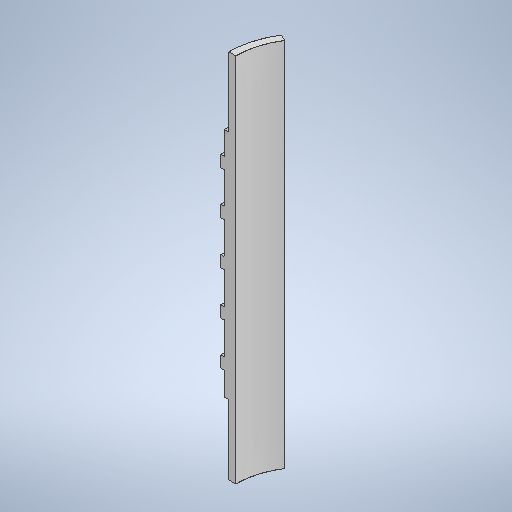
# Autodesk Inventor part: Bumper_V1
Saved by Autodesk Inventor 2025.2 (Build 292293000, 293)
## iProperties
Created: 2026-01-12
Part Number: Bumper_V1
Material: Generisch
Document SubType Name: Modeling
Designer: gassl
Density: 1 g/cm^3
Appearance: Vorgabe
Author: gassl
Autodesk Inventor part; units mm, degrees
ref_plane "YZ Plane" through (0, 0, 0) normal (1, 0, 0) x (0, 1, 0)
ref_plane "XZ Plane" through (0, 0, 0) normal (0, 1, 0) x (-1, 0, 0)
ref_plane "XY Plane" through (0, 0, 0) normal (0, 0, 1) x (1, 0, 0)
sketch "Skizze1" plane through (0, 0, 0) normal (0, 0, 1) x (1, 0, 0)
  arc A0 (-15, 25.9808) -> (-30, 0) centre (0, 0) ccw
  line L0 (-15, 25.9808) -> (-16.8174, 28.3932)
  line L1 (-30, 0) -> (-33, 0)
  arc A1 (-16.8174, 28.3932) -> (-33, 0) centre (0, 0) ccw
  constraints: 4 end point, 4 point on circle, 2 centre point, 1 coincident, 1 horizontal
extrude "Teil B1" add sketch "Skizze1" along normal blind 30
sketch "Skizze2" plane through (0, 0, 30) normal (0, 0, 1) x (1, 0, 0)
  arc A0 (-15, 25.9808) -> (-30, 0) centre (0, 0) ccw projected
  line L0 (-33, 0) -> (-30, 0) projected
  arc A1 (-15, 25.9808) -> (-30, 0) centre (0, 0) ccw
  arc A2 (-18.0278, 30) -> (-35, 0) centre (0, 0) ccw
  line L1 (-30, 0) -> (-35, 0)
  line L2 (-15, 25.9808) -> (-18.0278, 30)
  line L3 (-15, 25.9808) -> (-16.8174, 28.3932) projected
  dimension "d6" = 70
  constraints: 4 end point, 4 point on circle, 2 centre point, 1 coincident, 1 collinear, 1 point on line
  measures "d6" diameter of A2
extrude "Teil C1" add sketch "Skizze2" along normal blind 10
sketch "Skizze3" plane through (0, 0, 40) normal (0, 0, 1) x (1, 0, 0)
  arc A0 (-15, 25.9808) -> (-30, 0) centre (0, 0) ccw projected
  line L0 (-33, 0) -> (-30, 0) projected
  arc A1 (-15, 25.9808) -> (-30, 0) centre (0, 0) ccw
  arc A2 (-18.935, 31.2044) -> (-36.5, 0) centre (0, 0) ccw
  line L1 (-30, 0) -> (-36.5, 0)
  line L2 (-15, 25.9808) -> (-16.8174, 28.3932) projected
  line L3 (-15, 25.9808) -> (-18.935, 31.2044)
  dimension "d9" = 73
  constraints: 4 end point, 4 point on circle, 2 centre point, 1 coincident, 1 collinear, 1 horizontal
  measures "d9" diameter of A2
extrude "Teil D1" add sketch "Skizze3" along normal blind 5
sketch "Skizze4" plane through (0, 0, 45) normal (0, 0, 1) x (1, 0, 0)
  arc A0 (-18.0278, 30) -> (-35, 0) centre (0, 0) ccw
  arc A1 (-15, 25.9808) -> (-30, 0) centre (0, 0) ccw projected
  arc A2 (-15, 25.9808) -> (-30, 0) centre (0, 0) ccw
  line L0 (-16.8174, 28.3932) -> (-18.0278, 30) projected
  line L1 (-15, 25.9808) -> (-18.0278, 30)
  line L2 (-36.5, 0) -> (-35, 0) projected
  line L3 (-30, 0) -> (-35, 0)
  constraints: 4 end point, 4 point on circle, 2 centre point, 1 coincident, 1 collinear, 1 horizontal
extrude "Teil E1" add sketch "Skizze4" along normal blind 13.75
sketch "Skizze5" plane through (0, 0, 58.75) normal (0, 0, 1) x (1, 0, 0)
  arc A0 (-15, 25.9808) -> (-30, 0) centre (0, 0) ccw projected
  arc A1 (-15, 25.9808) -> (-30, 0) centre (0, 0) ccw
  arc A2 (-18.935, 31.2044) -> (-36.5, 0) centre (0, 0) ccw projected
  line L0 (-36.5, 0) -> (-35, 0) projected
  arc A3 (-18.935, 31.2044) -> (-36.5, 0) centre (0, 0) ccw
  line L1 (-33, 0) -> (-30, 0) projected
  line L2 (-36.5, 0) -> (-30, 0)
  line L3 (-15, 25.9808) -> (-18.935, 31.2044)
  point P0 (-15, 25.9808)
  constraints: 4 end point, 4 point on circle, 2 centre point, 1 collinear
extrude "Teil D2" add sketch "Skizze5" along normal blind 5
sketch "Skizze6" plane through (0, 0, 63.75) normal (0, 0, 1) x (1, 0, 0)
  line L0 (-33, 0) -> (-30, 0) projected
  arc A0 (-15, 25.9808) -> (-30, 0) centre (0, 0) ccw
  arc A1 (-18.0278, 30) -> (-35, 0) centre (0, 0) ccw projected
  arc A2 (-18.0278, 30) -> (-35, 0) centre (0, 0) ccw
  line L1 (-36.5, 0) -> (-35, 0) projected
  line L2 (-35, 0) -> (-30, 0)
  line L3 (-15, 25.9808) -> (-18.0278, 30)
  line L4 (-15, 25.9808) -> (-16.8174, 28.3932) projected
  constraints: 4 end point, 4 point on circle, 2 centre point, 2 collinear
extrude "Extrusion6" add sketch "Skizze6" along normal blind 13.75
sketch "Skizze7" plane through (0, 0, 77.5) normal (0, 0, 1) x (1, 0, 0)
  arc A0 (-15, 25.9808) -> (-30, 0) centre (0, 0) ccw projected
  line L0 (-33, 0) -> (-30, 0) projected
  arc A1 (-15, 25.9808) -> (-30, 0) centre (0, 0) ccw
  line L1 (-18.0278, 30) -> (-18.935, 31.2044) projected
  line L2 (-36.5, 0) -> (-35, 0) projected
  arc A2 (-18.935, 31.2044) -> (-36.5, 0) centre (0, 0) ccw
  line L3 (-36.5, 0) -> (-30, 0)
  line L4 (-15, 25.9808) -> (-16.8174, 28.3932) projected
  line L5 (-18.935, 31.2044) -> (-15, 25.9808)
  constraints: 4 end point, 4 point on circle, 2 centre point, 2 collinear
extrude "Extrusion7" add sketch "Skizze7" along normal blind 2.5
mirror "Spiegeln1" about plane through (-25.75, 15.6022, 80) normal (0, 0, 1)
sketch "Skizze8" plane through (-33, 0, 160) normal (0, 0, 1) x (1, 0, 0)
  arc A0 (18, 25.9808) -> (3, 0) centre (33, 0) ccw projected
  line L0 (3, 0) -> (13, 17.3205)
  line L1 (13, 17.3205) -> (4.1881, 22.4081)
  arc A1 (14.065, 31.2044) -> (-3.5, 0) centre (33, 0) ccw projected
  arc A2 (18, 25.9808) -> (9.8826, 19.1203) centre (33, 0) ccw
  arc A3 (14.065, 31.2044) -> (4.1881, 22.4081) centre (33, 0) ccw
  line L2 (14.065, 31.2044) -> (18, 25.9808)
  dimension "d21" = 20
  constraints: 6 end point, 6 point on circle, 2 centre point, 2 concentric, 1 perpendicular, 1 point on line
  measures "d21" distance of L0.start L0.end
extrude "Extrusion8" cut sketch "Skizze8" against normal through all contours A0 L1 A1 L2
sketch "Skizze9" plane through (-33, 0, 160) normal (0, 0, 1) x (1, 0, 0)
  line L0 (0, 0) -> (3, 0) projected
  arc A0 (9.8826, 19.1203) -> (3, 0) centre (33, 0) ccw projected
  arc A1 (3, 0) -> (7.8167, 16.3034) centre (-4.5602, 11.0968) ccw
  line L1 (7.8167, 16.3034) -> (1.9088, 19.1203)
  arc A2 (4.1881, 22.4081) -> (-3.5, 0) centre (33, 0) ccw projected
  line L2 (4.1881, 22.4081) -> (9.8826, 19.1203)
  arc A3 (4.1881, 22.4081) -> (1.9088, 19.1203) centre (33, 0) ccw
  arc A4 (9.8826, 19.1203) -> (7.8167, 16.3034) centre (33, 0) ccw
  dimension "d24" = 17
  constraints: 8 point on circle, 4 end point, 3 centre point, 3 concentric
  measures "d24" distance of L0.end L1.start
extrude "Extrusion9" cut sketch "Skizze9" against normal through all contours A0 L1 A2 L2
